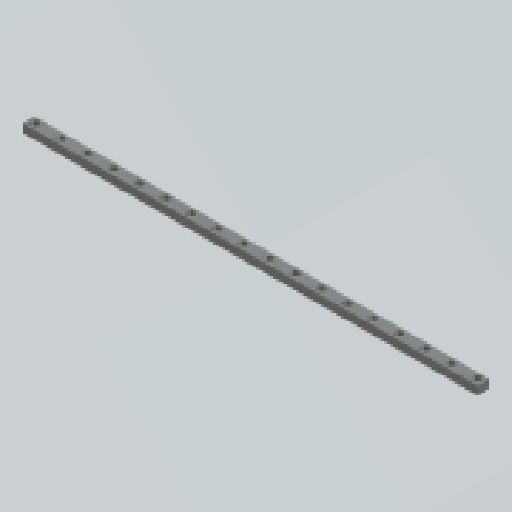
# Autodesk Inventor part: MGNR9_300mm
Saved by Autodesk Inventor 2023.2 (Build 272271000, 271)
## iProperties
Created: 2020-05-08
Part Number: MGNR9_300mm
Material: Stainless Steel
Document SubType Name: Modeling
Designer: Remo
Density: 8 g/cm^3
Appearance: Semi-Polished
Mass: 125.061 g
Surface Area: 106.128 cm^2
Volume: 15.6326 cm^3
Description: HIWIN MGNR9 Linear Rail
Author: Remo
Autodesk Inventor part; units mm, degrees
ref_plane "YZ Plane" through (0, 0, 0) normal (1, 0, 0) x (0, 1, 0)
ref_plane "XZ Plane" through (0, 0, 0) normal (0, 1, 0) x (-1, 0, 0)
ref_plane "XY Plane" through (0, 0, 0) normal (0, 0, 1) x (1, 0, 0)
sketch "Sketch1" plane through (0, 0, 0) normal (1, 0, 0) x (0, 1, 0)
  line L0 (-4.5, -3.25) -> (4.5, -3.25)
  line L1 (4.5, -3.25) -> (4.5, 3.25)
  line L2 (4.5, 3.25) -> (-4.5, 3.25)
  line L3 (-4.5, 3.25) -> (-4.5, -3.25)
  line L4 (-4.5, -3.25) -> (4.5, 3.25) construction
  line L5 (4.5, -3.25) -> (-4.5, 3.25) construction
  point P0 (0, 0)
  dimension "d0" = 9
  dimension "d1" = 6.5
  constraints: 12 end point, 2 midpoint, 2 parallel, 1 horizontal, 1 perpendicular
  measures "d0" distance of L0.start L0.end
  measures "d1" distance of L0.end L1.end
extrude "Extrusion1" add sketch "Sketch1" along normal blind 350
sketch "Sketch2" plane through (0, -4.5, 3.25) normal (0, 0, 1) x (1, 0, 0)
  line L0 (0, 9) -> (0, 0) projected
  line L1 (0, 9) -> (350, 9) projected
  point P0 (0, 4.5)
  point P1 (5, 4.5)
  point P2 (25, 4.5)
  point P3 (45, 4.5)
  point P4 (65, 4.5)
  point P5 (85, 4.5)
  point P6 (105, 4.5)
  point P7 (125, 4.5)
  point P8 (145, 4.5)
  point P9 (165, 4.5)
  point P10 (185, 4.5)
  point P11 (205, 4.5)
  point P12 (225, 4.5)
  point P13 (245, 4.5)
  point P14 (265, 4.5)
  point P15 (285, 4.5)
  point P16 (305, 4.5)
  point P17 (325, 4.5)
  point P18 (345, 4.5)
  point P19 (365, 4.5)
  point P20 (385, 4.5)
  point P21 (405, 4.5)
  point P22 (425, 4.5)
  point P23 (445, 4.5)
  point P24 (465, 4.5)
  point P25 (485, 4.5)
  point P26 (505, 4.5)
  point P27 (525, 4.5)
  point P28 (545, 4.5)
  point P29 (565, 4.5)
  dimension "d4" = 5
  dimension "d5" = 4.5
  dimension "d8" = 20
  constraints: 1 horizontal, 28 other
  measures "d4" distance from line of L0 point (5, 4.5)
  measures "d5" distance from line of L1 point (5, 4.5)
  measures "d8" distance of point (5, 4.5) point (25, 4.5)
hole "Hole1" at (5, 0, 3.25) at (25, 0, 3.25) at (45, 0, 3.25) at (65, 0, 3.25) at (85, 0, 3.25) at (105, 0, 3.25) at (125, 0, 3.25) at (145, 0, 3.25) at (165, 0, 3.25) at (185, 0, 3.25) at (205, 0, 3.25) at (225, 0, 3.25) at (245, 0, 3.25) at (265, 0, 3.25) at (285, 0, 3.25) at (305, 0, 3.25) at (325, 0, 3.25) at (345, 0, 3.25) at (365, 0, 3.25) at (385, 0, 3.25) at (405, 0, 3.25) at (425, 0, 3.25) at (445, 0, 3.25) at (465, 0, 3.25) at (485, 0, 3.25) at (505, 0, 3.25) at (525, 0, 3.25) at (545, 0, 3.25) at (565, 0, 3.25) direction (0, 0, -1) diameter 3.5 depth 8 tip angle 118 counterbore diameter 6 counterbore depth 3.5
body "Solid1"
